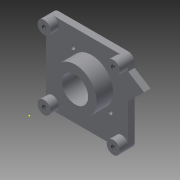
# Autodesk Inventor part: Face Plate
Saved by Autodesk Inventor 2015 (Build 190159000, 159)
## iProperties
Created: 2016-02-13
Part Number: Face Plate
Material: Generic
Document SubType Name: Modeling
Designer: Owner
Density: 1 g/cm^3
Appearance: Default
Mass: 6.92583 g
Surface Area: 50.6167 cm^2
Volume: 6.92583 cm^3
Author: Owner
Autodesk Inventor part; units mm, degrees
ref_plane "YZ Plane" through (0, 0, 0) normal (1, 0, 0) x (0, 1, 0)
ref_plane "XZ Plane" through (0, 0, 0) normal (0, 1, 0) x (-1, 0, 0)
ref_plane "XY Plane" through (0, 0, 0) normal (0, 0, 1) x (1, 0, 0)
sketch "Sketch1" plane through (0, 0, 0) normal (0, 0, 1) x (1, 0, 0)
  line L0 (0, 0) -> (40.005, 0)
  line L1 (40.005, 0) -> (40.005, 40.005)
  line L2 (40.005, 40.005) -> (0, 40.005)
  line L3 (0, 40.005) -> (0, 0)
  line L4 (40.005, 40.005) -> (40.005, 34.6202)
  line L5 (40.005, 34.6202) -> (47.7434, 29.7489)
  line L6 (40.005, 34.6202) -> (49.149, 34.6202) construction
  line L7 (47.7434, 29.7489) -> (40.005, 22.0414)
  dimension "d0" = 40.005
  dimension "d1" = 40.005
  dimension "d2" = 5.3848
  dimension "d3" = 9.144
  dimension "d5" = 10.922
  dimension "d6" = 57.81
  constraints: 16 end point, 2 horizontal, 2 parallel, 2 point on line, 1 equal length, 1 perpendicular
  measures "d0" distance of L2.end L1.end
  measures "d1" distance of L0.end L1.end
  measures "d2" distance of L1.end L4.end
  measures "d3" distance of L4.end L5.end
  measures "d5" distance of L5.end L7.end
  measures "d6" angle of L5 L1
extrude "Extrusion1" add sketch "Sketch1" along normal blind 3.175
fillet "Fillet1" radius 3.175 4 edges at (0, 0, 1.5875) (0, 40.005, 1.5875) (40.005, 40.005, 1.5875) (40.005, 0, 1.5875)
sketch "Sketch2" plane through (0, 0, 3.175) normal (0, 0, 1) x (1, 0, 0)
  line L0 (0, 36.83) -> (0, 3.175) projected
  line L1 (3.175, 0) -> (36.83, 0) projected
  line L2 (40.005, 3.175) -> (40.005, 22.0414) projected
  line L3 (36.83, 40.005) -> (3.175, 40.005) projected
  circle A0 centre (3.175, 3.175) radius 3.169
  circle A1 centre (36.83, 3.175) radius 3.175
  circle A2 centre (36.83, 36.83) radius 3.175
  circle A3 centre (3.175, 36.83) radius 3.1755
  point P0 (0, 0)
  dimension "d10" = 6.35
  constraints: 4 centre point
  measures "d10" diameter of A2
extrude "Extrusion2" add sketch "Sketch2" along normal blind 4.064
sketch "Sketch3" plane through (3.175, 36.83, 7.239) normal (0, 0, 1) x (1, 0, 0)
  circle A0 centre (0, 0) radius 3.1755 projected
  circle A1 centre (33.655, 0) radius 3.175 projected
  circle A2 centre (33.655, -33.655) radius 3.175 projected
  circle A3 centre (0, -33.655) radius 3.169 projected
  point P0 (-3.175, -36.83)
hole "Hole1" at (3.175, 36.83, 7.239) at (36.83, 36.83, 7.239) at (36.83, 3.175, 7.239) at (3.175, 3.175, 7.239) direction (0, 0, -1) diameter 2.159 end through all
sketch "Sketch4" plane through (0, 0, 3.175) normal (0, 0, 1) x (1, 0, 0)
  arc A0 (0, 3.175) -> (3.175, 0) centre (3.175, 3.175) ccw projected
  circle A1 centre (3.175, 3.175) radius 3.169 projected
  line L0 (0, 0) -> (22.2172, 22.2172)
  line L1 (0, 0) -> (31.4198, 0) construction
  circle A2 centre (22.2172, 22.2172) radius 10.4902
  dimension "d20" = 31.4198
  dimension "d21" = 45
  dimension "d22" = 20.9804
  constraints: 4 end point, 1 centre point, 1 coincident, 1 equal length, 1 horizontal
  measures "d20" distance of L0.start L0.end
  measures "d21" angle of L1 L0
  measures "d22" diameter of A2
extrude "Extrusion3" add sketch "Sketch4" along normal blind 8.001 contours A2
sketch "Sketch5" plane through (22.2172, 22.2172, 11.176) normal (0, 0, 1) x (1, 0, 0)
  point P0 (-22.2172, -22.2172)
sketch "Sketch6" plane through (22.2172, 22.2172, 11.176) normal (0, 0, 1) x (1, 0, 0)
  circle A0 centre (0, 0) radius 6.35
  point P0 (-22.2172, -22.2172)
  dimension "d25" = 12.7
  constraints: 1 centre point
  measures "d25" diameter of A0
extrude "Extrusion4" cut sketch "Sketch6" against normal through all
sketch "Sketch7" plane through (0, 0, 3.175) normal (0, 0, 1) x (1, 0, 0)
  circle A0 centre (22.2172, 22.2172) radius 6.35 projected
  circle A1 centre (22.2172, 22.2172) radius 10.4902 projected
  line L0 (13.1318, 31.3182) -> (13.1318, 13.1318) construction
  line L1 (13.1318, 13.1318) -> (31.3182, 13.1318) construction
  line L2 (13.1318, 31.3182) -> (31.3182, 31.3182) construction
  line L3 (31.3182, 31.3182) -> (31.3182, 13.1318) construction
  point P0 (0, 0)
  dimension "d30" = 18.1864
  constraints: 8 end point, 2 perpendicular, 1 horizontal
  measures "d30" distance of L0.start L0.end
hole "Hole2" at (13.1318, 13.1318, 3.175) at (31.3182, 31.3182, 3.175) at (13.1318, 31.3182, 3.175) at (31.3182, 13.1318, 3.175) direction (0, 0, -1) diameter 2.032 end through all
body "Solid1"
